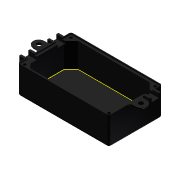
# Autodesk Inventor part: корпус
Saved by Autodesk Inventor 2012 (Build 160160000, 160)
## iProperties
Created: 2009-09-07
Part Number: корпус
Material: По умолчанию
Document SubType Name: Обычные детали
Designer: toma
Density: 1 g/cm^3
Mass: 11.7492 g
Surface Area: 128.19 cm^2
Volume: 11.7492 cm^3
Sheet Metal Rule: По умолчанию_мм
Author: toma
Autodesk Inventor part; units mm, degrees
ref_plane "YZ Plane" through (0, 0, 0) normal (1, 0, 0) x (0, 1, 0)
ref_plane "XZ Plane" through (0, 0, 0) normal (0, 1, 0) x (-1, 0, 0)
ref_plane "XY Plane" through (0, 0, 0) normal (0, 0, 1) x (1, 0, 0)
sketch "Эскиз1" plane through (0, 0, 0) normal (0, 0, 1) x (1, 0, 0)
  line L0 (29, 24) -> (-36, 24)
  line L1 (-36, -14) -> (29, -14)
  line L2 (29, -14) -> (29, 24)
  line L3 (-36, -14) -> (-36, 24)
  dimension "d0" = 65
  dimension "d1" = 65
  constraints: 8 end point, 1 horizontal, 1 parallel, 1 perpendicular
  measures "d0" distance of L0.start L0.end
  measures "d1" distance of L1.start L1.end
extrude "Выдавливание1" add sketch "Эскиз1" along normal blind 1.5
sketch "Эскиз7" plane through (0, 0, 0) normal (0, 0, -1) x (-1, 0, 0)
  line L0 (-29, 24) -> (36, 24) projected
  line L1 (36, -14) -> (-29, -14) projected
  line L2 (-29, -14) -> (36, -14)
  line L3 (36, -14) -> (36, 24)
  line L4 (36, 24) -> (-29, 24)
  line L5 (-29, 24) -> (-29, -14)
  line L6 (-22, -12) -> (29, -12)
  line L7 (34, -7) -> (34, 17)
  line L8 (29, 22) -> (-22, 22)
  line L9 (-27, 17) -> (-27, -7)
  line L10 (-27, 17) -> (-22, 22)
  line L11 (29, 22) -> (34, 17)
  line L12 (34, -7) -> (29, -12)
  line L13 (-22, -12) -> (-27, -7)
  point P0 (36, -9)
  point P1 (-27, -12)
  point P2 (34, 22)
  point P3 (34, -12)
  point P4 (-27, 22)
  dimension "d77" = 2
  dimension "d78" = 2
  dimension "d79" = 2
  dimension "d80" = 2
  dimension "d81" = 5
  dimension "d82" = 45
  dimension "d83" = 5
  dimension "d84" = 45
  dimension "d85" = 5
  dimension "d86" = 45
  dimension "d87" = 5
  dimension "d88" = 45
  constraints: 24 end point, 8 point on line, 4 parallel, 2 horizontal, 2 perpendicular
  measures "d77" distance between parallel lines of L8 L0
  measures "d78" distance between parallel lines of L5 L9
  measures "d79" distance between parallel lines of L1 L6
  measures "d80" distance from line of point (36, -9) L7
  measures "d81" distance of L9.start point (-27, 22)
  measures "d82" angle of L9 L10
  measures "d83" distance of L8.start point (34, 22)
  measures "d84" angle of L8 L11
  measures "d85" distance of L7.start point (34, -12)
  measures "d86" angle of L7 L12
  measures "d87" distance of L6.start point (-27, -12)
  measures "d88" angle of L6 L13
extrude "Выдавливание5" add sketch "Эскиз7" against normal blind 20
sketch "Эскиз10" plane through (0, 0, 1.5) normal (0, 0, 1) x (1, 0, 0)
  line L0 (27, -7) -> (27, 17) projected
  line L1 (27, 17) -> (22, 22) projected
  line L2 (22, 22) -> (-29, 22) projected
  line L3 (-29, 22) -> (-34, 17) projected
  line L4 (-34, 17) -> (-34, -7) projected
  line L5 (-34, -7) -> (-29, -12) projected
  line L6 (-29, -12) -> (22, -12) projected
  line L7 (22, -12) -> (27, -7) projected
sketch "Эскиз12" plane through (0, 0, 20) normal (0, 0, 1) x (1, 0, 0)
  line L0 (29, 24) -> (29, -14) projected
  line L1 (-36, -14) -> (-36, 24) projected
  line L2 (29, -14) -> (-36, -14) projected
  line L3 (-36, 19) -> (-40, 19)
  line L4 (-40, 19) -> (-40, 11)
  line L5 (-40, 11) -> (-36, 11)
  line L6 (-36, 11) -> (-36, 19)
  line L7 (-36, -1) -> (-40, -1)
  line L8 (-40, -1) -> (-40, -9)
  line L9 (-40, -9) -> (-36, -9)
  line L10 (-36, -1) -> (-36, -9)
  line L11 (29, 19) -> (33, 19)
  line L12 (33, 19) -> (33, 11)
  line L13 (33, 11) -> (29, 11)
  line L14 (29, 11) -> (29, 19)
  constraints: 24 end point, 9 perpendicular, 6 point on line, 2 collinear, 1 parallel
extrude "Выдавливание8" add sketch "Эскиз12" against normal blind 4.5
sketch "Эскиз13" plane through (-40, 11, 20) normal (-1, 0, 0) x (0, 0, 1)
  line L0 (-4.5, 8) -> (-4.5, 0) projected
  line L1 (0, 0) -> (-4.5, 0) projected
  line L2 (0, 8) -> (-4.5, 8) projected
  line L3 (-3, 1.5) -> (1, 1.5)
  line L4 (1, 1.5) -> (1, 6.5)
  line L5 (1, 6.5) -> (-3, 6.5)
  line L6 (-3, 6.5) -> (-3, 1.5)
  dimension "d100" = 1.5
  dimension "d101" = 1.5
  dimension "d102" = 1.5
  constraints: 8 end point, 2 parallel, 1 horizontal, 1 perpendicular
  measures "d100" distance between parallel lines of L2 L5
  measures "d101" distance between parallel lines of L0 L6
  measures "d102" distance between parallel lines of L1 L3
extrude "Выдавливание9" cut sketch "Эскиз13" against normal through all
sketch "Эскиз14" plane through (-40, -9, 20) normal (-1, 0, 0) x (0, 0, 1)
  line L0 (-4.5, 8) -> (-4.5, 0) projected
  line L1 (0, 0) -> (-4.5, 0) projected
  line L2 (0, 8) -> (-4.5, 8) projected
  line L3 (-3, 6.5) -> (1, 6.5)
  line L4 (1, 6.5) -> (1, 1.5)
  line L5 (1, 1.5) -> (-3, 1.5)
  line L6 (-3, 1.5) -> (-3, 6.5)
  dimension "d105" = 1.5
  dimension "d106" = 1.5
  dimension "d107" = 1.5
  constraints: 8 end point, 2 parallel, 1 horizontal, 1 perpendicular
  measures "d105" distance between parallel lines of L2 L3
  measures "d106" distance between parallel lines of L0 L6
  measures "d107" distance between parallel lines of L1 L5
extrude "Выдавливание10" cut sketch "Эскиз14" against normal blind 10
sketch "Эскиз15" plane through (0, 0, 1.5) normal (0, 0, 1) x (1, 0, 0)
  line L0 (27, -7) -> (27, 17) projected
  line L1 (27, 17) -> (22, 22) projected
  line L2 (22, 22) -> (-29, 22) projected
  line L3 (-29, 22) -> (-34, 17) projected
  line L4 (-34, 17) -> (-34, -7) projected
  line L5 (-34, -7) -> (-29, -12) projected
  line L6 (-29, -12) -> (22, -12) projected
  line L7 (22, -12) -> (27, -7) projected
  line L8 (-43.8933, 5) -> (-43.8933, 5)
  line L9 (-36, 11) -> (-36, 11)
  line L10 (-36, -1) -> (-36, -1)
  constraints: 6 end point
sketch "Эскиз16" plane through (0, 0, 20) normal (0, 0, 1) x (1, 0, 0)
  line L0 (-36, -1) -> (-36, 11) projected
  line L1 (-40, -1) -> (-40, -2.5) projected
  line L2 (-38, 9) -> (-40, 9)
  line L3 (-44, 5) -> (-44, 5)
  line L4 (-40, 1) -> (-38, 1)
  line L5 (-36, 11) -> (-36, 11)
  arc A0 (-40, 9) -> (-44, 5) centre (-40, 5) ccw
  arc A1 (-44, 5) -> (-40, 1) centre (-40, 5) ccw
  arc A2 (-38, 9) -> (-36, 11) centre (-38, 11) ccw
  line L6 (-36, -1) -> (-36, -1)
  arc A3 (-36, -1) -> (-38, 1) centre (-38, -1) ccw
  point P0 (-36, 9)
  point P1 (-36, 1)
  dimension "d113" = 4
  dimension "d114" = 2
  dimension "d115" = 2
  constraints: 10 end point, 8 point on circle, 8 tangent, 6 point on line, 4 centre point, 4 perpendicular, 1 collinear, 1 concentric
  measures "d113" radius of A0
  measures "d114" radius of A2
  measures "d115" radius of A3
sketch "Эскиз17" plane through (0, 0, 20) normal (0, 0, 1) x (1, 0, 0)
  line L0 (29, 11) -> (29, -14) projected
  line L1 (22, -12) -> (-29, -12) projected
  line L2 (31, 9) -> (33, 9)
  line L3 (37, 5) -> (37, 5)
  line L4 (33, 1) -> (31, 1)
  line L5 (29, 11) -> (29, 11)
  line L6 (29, -1) -> (29, -1)
  line L7 (29, 1) -> (29, 9)
  arc A0 (37, 5) -> (33, 9) centre (33, 5) ccw
  arc A1 (33, 1) -> (37, 5) centre (33, 5) ccw
  arc A2 (29, 11) -> (31, 9) centre (31, 11) ccw
  arc A3 (31, 1) -> (29, -1) centre (31, -1) ccw
  dimension "d116" = 4
  dimension "d117" = 2
  dimension "d118" = 2
  constraints: 12 end point, 8 point on circle, 8 tangent, 7 point on line, 4 centre point, 2 collinear, 2 perpendicular, 1 concentric, 1 parallel
  measures "d116" radius of A0
  measures "d117" radius of A2
  measures "d118" radius of A3
extrude "Выдавливание11" add sketch "Эскиз16" against normal blind 1.5
extrude "Выдавливание12" add sketch "Эскиз17" against normal blind 1.5
sketch "Эскиз18" plane through (0, 0, 1.5) normal (0, 0, 1) x (1, 0, 0)
  line L0 (27, -7) -> (27, 17) projected
  line L1 (27, 17) -> (22, 22) projected
  line L2 (22, 22) -> (-29, 22) projected
  line L3 (-29, 22) -> (-34, 17) projected
  line L4 (-34, 17) -> (-34, -7) projected
  line L5 (-34, -7) -> (-29, -12) projected
  line L6 (-29, -12) -> (22, -12) projected
  line L7 (22, -12) -> (27, -7) projected
sketch "Эскиз19" plane through (0, 0, 20) normal (0, 0, 1) x (1, 0, 0)
  line L0 (29, 24) -> (29, 19) projected
  line L1 (-36, 24) -> (29, 24) projected
  line L2 (-36, 19) -> (-36, 24) projected
  line L3 (-35.5, -13.5) -> (28.5, -13.5)
  line L4 (28.5, -13.5) -> (28.5, 23.5)
  line L5 (28.5, 23.5) -> (-35.5, 23.5)
  line L6 (-35.5, 23.5) -> (-35.5, -13.5)
  line L7 (29, -14) -> (-36, -14) projected
  dimension "d123" = 0.5
  dimension "d124" = 0.5
  dimension "d125" = 0.5
  dimension "d126" = 0.5
  constraints: 8 end point, 2 parallel, 1 horizontal, 1 perpendicular
  measures "d123" distance between parallel lines of L6 L2
  measures "d124" distance from line of L4.end L0
  measures "d125" distance between parallel lines of L3 L7
  measures "d126" distance between parallel lines of L1 L5
extrude "Выдавливание13" cut sketch "Эскиз19" against normal blind 1
sketch "Эскиз20" plane through (0, 0, 20) normal (0, 0, 1) x (1, 0, 0)
  arc A0 (-40, 9) -> (-40, 1) centre (-40, 5) ccw projected
  line L0 (-40, -2.5) -> (-35.5, -2.5) projected
  line L1 (-40, 5) -> (33, 5) construction
  point P0 (-39.8, 5)
  point P1 (32.8, 5)
  dimension "d129" = 0.2
  dimension "d130" = 72.6
  constraints: 2 end point, 2 point on line, 1 parallel
  measures "d129" distance of point (-39.8, 5) L1.start
  measures "d130" distance of point (32.8, 5) point (-39.8, 5)
hole "Отверстие1" at (-39.8, 5, 20) at (32.8, 5, 20) direction (0, 0, -1) diameter 3.2 end through all
sketch "Эскиз21" plane through (0, 0, 19) normal (0, 0, 1) x (1, 0, 0)
  line L0 (-33.5, -11.5) -> (26.5, -11.5) construction
  line L1 (26.5, -11.5) -> (26.5, 21.5) construction
  line L2 (26.5, 21.5) -> (-33.5, 21.5) construction
  line L3 (-33.5, 21.5) -> (-33.5, -11.5) construction
  line L4 (-36, 19) -> (-36, 24) construction
  line L5 (-36, 24) -> (29, 24) construction
  dimension "d138" = 60
  dimension "d139" = 33
  dimension "d140" = 2.5
  dimension "d141" = 2.5
  constraints: 8 end point, 4 coincident, 2 parallel, 1 horizontal, 1 perpendicular
  measures "d138" distance between parallel lines of L1 L3
  measures "d139" distance between parallel lines of L0 L2
  measures "d140" distance between parallel lines of L3 L4
  measures "d141" distance between parallel lines of L5 L2
hole "Отверстие2" at (-33.5, 21.5, 19) at (-33.5, -11.5, 19) at (26.5, 21.5, 19) at (26.5, -11.5, 19) direction (0, 0, -1) diameter 2 depth 3.2 tip angle 118
fillet "Сопряжение4" radius 1.5 8 edges at (-3.5, -14, 0) (-36, 5, 0) (-36, -14, 10) (-36, 24, 10) (29, -14, 10) (29, 5, 0) (29, 24, 10) (-3.5, 24, 0)
fillet "Сопряжение5" radius 1.5 10 edges at (37, 5, 18.5) (32, 9, 18.5) (29.5858, 9.5858, 18.5) (32, 1, 18.5) (29.5858, 0.4142, 18.5) (-44, 5, 18.5) (-39, 1, 18.5) (-36.5858, 0.4142, 18.5) (-39, 9, 18.5) (-36.5858, 9.5858, 18.5)
fillet "Сопряжение6" radius 0.25 15 edges at (-38, -9, 15.5) (-40, -5, 15.5) (-38, -1, 15.5) (-40, -9, 17.75) (-40, -1, 17.75) (-40, 19, 17.75) (-38, 19, 15.5) (-40, 15, 15.5) (-38, 11, 15.5) (-40, 11, 17.75) (33, 19, 17.75) (33, 15, 15.5) (33, 11, 17.75) (31, 11, 15.5) (31, 19, 15.5)
fillet "Сопряжение7" radius 0.5 4 edges at (28.5, 23.5, 19.5) (28.5, -13.5, 19.5) (-35.5, 23.5, 19.5) (-35.5, -13.5, 19.5)
equation "\"d83\" = d81"
equation "\"d84\" = d82"
equation "\"d85\" = d81"
equation "\"d86\" = d82"
equation "\"d87\" = d81"
equation "\"d88\" = d82"
equation "\"Радиус_гибки\" = Толщина"
equation "\"Ширина_просечки\" = Толщина"
equation "\"Глубина_просечки\" = 0.5 * Толщина"
equation "\"Размер_высечки\" = 4 * Толщина"
equation "\"Мин_остаток\" = 2 * Толщина"
equation "\"Радиус_перехода\" = Радиус_гибки"
equation "\"Радиус_Якоби\" = Радиус_гибки"
equation "\"Размер_зазора\" = Толщина"
equation "\"Толщина\" = 0.5"
